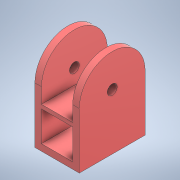
# Autodesk Inventor part: REDONDA
Saved by Autodesk Inventor 2022.6 (Build 266554000, 554)
## iProperties
Created: 2025-02-20
Part Number: REDONDA
Material: Genérico
Document SubType Name: Modeling
Designer: Johan Gutiérrez
Density: 1 g/cm^3
Appearance: Valor por defecto
Author: Johan Gutiérrez
Autodesk Inventor part; units mm, degrees
ref_plane "YZ Plane" through (0, 0, 0) normal (1, 0, 0) x (0, 1, 0)
ref_plane "XZ Plane" through (0, 0, 0) normal (0, 1, 0) x (-1, 0, 0)
ref_plane "XY Plane" through (0, 0, 0) normal (0, 0, 1) x (1, 0, 0)
sketch "Boceto1" plane through (0, 0, 0) normal (0, 1, 0) x (-1, 0, 0)
  line L0 (0, 0) -> (27, 0)
  line L1 (27, 0) -> (27, -40)
  line L2 (27, -40) -> (0, -40)
  line L3 (0, -40) -> (0, 0)
  dimension "d0" = 27
  dimension "d1" = 40
  constraints: 8 end point, 2 parallel, 1 horizontal, 1 perpendicular
  measures "d0" distance of L1.end L2.end
  measures "d1" distance of L0.end L1.end
extrude "Extrusión1" add sketch "Boceto1" along normal blind 54
sketch "Boceto2" plane through (-27, 0, 0) normal (0, 0, 1) x (1, 0, 0)
  line L0 (4, 4) -> (23, 4)
  line L1 (23, 4) -> (23, 22.3365)
  line L2 (23, 22.3365) -> (4, 22.3365)
  line L3 (4, 22.3365) -> (4, 4)
  line L4 (0, 0) -> (27, 0) projected
  line L5 (27, 0) -> (27, 54) projected
  line L6 (0, 54) -> (27, 54) projected
  line L7 (0, 0) -> (0, 54) projected
  line L8 (27, 54) -> (0, 54) projected
  line L9 (4, 24.7292) -> (23, 24.7292)
  line L10 (23, 24.7292) -> (23, 54)
  line L11 (23, 54) -> (4, 54)
  line L12 (4, 54) -> (4, 24.7292)
  point P0 (4, 54)
  dimension "d4" = 4
  dimension "d5" = 4
  dimension "d6" = 4
  constraints: 16 end point, 4 parallel, 2 horizontal, 2 perpendicular, 1 point on line
  measures "d4" distance between parallel lines of L4 L0
  measures "d5" distance between parallel lines of L5 L1
  measures "d6" distance between parallel lines of L7 L3
extrude "Extrusión2" cut sketch "Boceto2" against normal blind 54 contours L3 L2 L1 L0 | L6 L10 L9 L12
sketch "Boceto3" plane through (0, 0, 0) normal (1, 0, 0) x (0, 0, -1)
  line L0 (0, 0) -> (40, 0) projected
  line L1 (40, 0) -> (40, 54) projected
  line L2 (0, 54) -> (40, 54) projected
  line L3 (0, 0) -> (0, 54) projected
  line L4 (0, 54) -> (40, 54) projected
  line L5 (20, 54) -> (20, 34)
  circle A0 centre (20, 34) radius 3
  dimension "d9" = 20
  dimension "d10" = 6
  constraints: 2 end point, 1 centre point, 1 coincident, 1 midpoint, 1 vertical
  measures "d9" distance of L5.start L5.end
  measures "d10" diameter of A0
extrude "Extrusión3" cut sketch "Boceto3" against normal blind 54 contours A0
sketch "Boceto4" plane through (0, 0, 0) normal (1, 0, 0) x (0, 0, -1)
  circle A0 centre (20, 34) radius 3 projected
  line L0 (0, 0) -> (40, 0) projected
  line L1 (40, 0) -> (40, 54) projected
  line L2 (0, 54) -> (40, 54) projected
  line L3 (0, 0) -> (0, 54) projected
  line L4 (40, 54) -> (0, 54) projected
  circle A1 centre (20, 34) radius 3 projected
  circle A2 centre (20, 34) radius 20
  point P0 (0, 34)
  point P1 (20, 54)
  point P2 (40, 34)
  constraints: 1 centre point, 1 coincident
extrude "Extrusión4" cut sketch "Boceto4" against normal blind 54 contours L3 L2 A2 | A2 L2 L1
